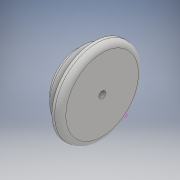
# Autodesk Inventor part: tapa carcasa camara
Saved by Autodesk Inventor 2018 (Build 220112000, 112)
## iProperties
Created: 2018-02-25
Part Number: tapa carcasa camara
Material: Genérico
Document SubType Name: Modeling
Designer: ivanb
Density: 1 g/cm^3
Appearance: Valor por defecto
Author: ivanb
Autodesk Inventor part; units mm, degrees
ref_plane "YZ Plane" through (0, 0, 0) normal (1, 0, 0) x (0, 1, 0)
ref_plane "XZ Plane" through (0, 0, 0) normal (0, 1, 0) x (-1, 0, 0)
ref_plane "XY Plane" through (0, 0, 0) normal (0, 0, 1) x (1, 0, 0)
sketch "Boceto1" plane through (0, 0, 0) normal (1, 0, 0) x (0, 1, 0)
  circle A0 centre (0, 0) radius 5.9
  dimension "d0" = 11.8
  constraints: 1 centre point, 1 coincident
  measures "d0" diameter of A0
extrude "Extrusión1" add sketch "Boceto1" along normal blind 3
sketch "Boceto2" plane through (3, 0, 0) normal (1, 0, 0) x (0, 0, -1)
  circle A0 centre (0, 0) radius 7.5
  dimension "d3" = 15
  constraints: 1 centre point, 1 coincident
  measures "d3" diameter of A0
extrude "Extrusión2" add sketch "Boceto2" against normal blind 1.5
sketch "Boceto3" plane through (0, 0, 0) normal (-1, 0, 0) x (0, 0, 1)
  circle A0 centre (0, 0) radius 4.75
  dimension "d6" = 9.5
  constraints: 1 centre point, 1 coincident
  measures "d6" diameter of A0
extrude "Extrusión3" cut sketch "Boceto3" against normal blind 2
fillet "Empalme1" radius 1 1 edges at (3, 0, 7.5)
sketch "Boceto4" plane through (3, 0, 0) normal (1, 0, 0) x (0, 0, -1)
  circle A0 centre (0, 0) radius 0.6
  dimension "d13" = 1.2
  constraints: 1 centre point, 1 coincident
  measures "d13" diameter of A0
extrude "Extrusión4" cut sketch "Boceto4" against normal blind 10
sketch "Boceto5" plane through (0, 0, 0) normal (-1, 0, 0) x (0, 0, 1)
  circle A0 centre (0, 0) radius 5.9
  circle A1 centre (0, 0) radius 5.9 projected
  circle A2 centre (0, 0) radius 4.75
  constraints: 2 centre point, 2 coincident
extrude "Extrusión5" add sketch "Boceto5" along normal blind 1.5
chamfer "Chaflán2" distance 1 angle 45 1 edges at (-1.5, 0, -5.9)
